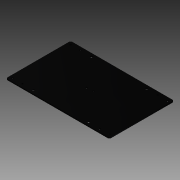
# Autodesk Inventor part: y-carriage
Saved by Autodesk Inventor 2014 (Build 180170000, 170)
## iProperties
Created: 2013-07-12
Part Number: y-carriage
Material: Steel, Mild
Document SubType Name: Modeling
Designer: Edward
Density: 7.86 g/cm^3
Appearance: Smooth - Black
Author: Edward
Autodesk Inventor part; units mm, degrees
ref_plane "YZ Plane" through (0, 0, 0) normal (1, 0, 0) x (0, 1, 0)
ref_plane "XZ Plane" through (0, 0, 0) normal (0, 1, 0) x (-1, 0, 0)
ref_plane "XY Plane" through (0, 0, 0) normal (0, 0, 1) x (1, 0, 0)
sketch "Sketch1" plane through (0, 0, 0) normal (0, 0, 1) x (1, 0, 0)
  line L0 (-160, 100) -> (160, 100)
  line L1 (160, 100) -> (160, -100)
  line L2 (160, -100) -> (-160, -100)
  line L3 (-160, -100) -> (-160, 100)
  point P0 (0, 0)
  dimension "d0" = 320
  dimension "d1" = 200
  dimension "d2" = 160
  dimension "d3" = 100
  constraints: 8 end point, 2 parallel, 1 horizontal, 1 perpendicular
  measures "d0" distance of L1.end L2.end
  measures "d1" distance of L0.end L1.end
  measures "d2" distance from line of point (0, 0) L3
  measures "d3" distance from line of L0 point (0, 0)
extrude "Extrusion1" add sketch "Sketch1" along normal blind 3.4163
sketch "Sketch2" plane through (0, 0, 3.4163) normal (0, 0, 1) x (1, 0, 0)
  line L0 (160, 100) -> (-160, 100) projected
  line L1 (-160, 100) -> (-160, -100) projected
  line L2 (-160, -100) -> (160, -100) projected
  line L3 (160, -100) -> (160, 100) projected
  circle A0 centre (-150, -90) radius 2.75
  circle A1 centre (-150, 90) radius 2.75
  circle A2 centre (-85.4, 90) radius 3.58
  circle A3 centre (-85.4, -90) radius 3.58
  circle A4 centre (85.4, 90) radius 3.58
  circle A5 centre (150, 90) radius 2.75
  circle A6 centre (85.4, -90) radius 3.58
  circle A7 centre (150, -90) radius 2.75
  point P0 (0, 0)
  dimension "d6" = 5.5
  dimension "d7" = 5.5
  dimension "d8" = 7.16
  dimension "d9" = 7.16
  dimension "d10" = 7.16
  dimension "d11" = 5.5
  dimension "d12" = 7.16
  dimension "d13" = 5.5
  dimension "d14" = 10
  dimension "d15" = 10
  dimension "d16" = 64.6
  dimension "d17" = 10
  dimension "d18" = 64.6
  dimension "d19" = 10
  dimension "d20" = 10
  dimension "d21" = 10
  dimension "d22" = 10
  dimension "d23" = 10
  dimension "d24" = 10
  dimension "d25" = 10
  dimension "d26" = 10
  dimension "d27" = 64.6
  dimension "d28" = 64.6
  dimension "d29" = 10
  constraints: 8 centre point
  measures "d6" diameter of A0
  measures "d7" diameter of A1
  measures "d8" diameter of A2
  measures "d9" diameter of A3
  measures "d10" diameter of A4
  measures "d11" diameter of A5
  measures "d12" diameter of A6
  measures "d13" diameter of A7
  measures "d14" distance from line of L2 A0.centre
  measures "d15" distance from line of L1 A0.centre
  measures "d16" distance of A3.centre A0.centre
  measures "d17" distance from line of L2 A3.centre
  measures "d18" distance of A2.centre A1.centre
  measures "d19" distance from line of L0 A1.centre
  measures "d20" distance from line of L1 A1.centre
  measures "d21" distance from line of L0 A2.centre
  measures "d22" distance from line of L2 A7.centre
  measures "d23" distance from line of L3 A7.centre
  measures "d24" distance from line of L3 A5.centre
  measures "d25" distance from line of L0 A5.centre
  measures "d26" distance from line of L0 A4.centre
  measures "d27" distance of A5.centre A4.centre
  measures "d28" distance of A6.centre A7.centre
  measures "d29" distance from line of L2 A6.centre
extrude "Extrusion2" cut sketch "Sketch2" against normal through all contours A0 | A1 | A2 | A3 | A4 | A5 | A6 | A7
fillet "Fillet1" radius 5 4 edges at (-160, -100, 1.7082) (-160, 100, 1.7082) (160, 100, 1.7082) (160, -100, 1.7082)
sketch "Sketch3" plane through (0, 0, 0) normal (0, 0, -1) x (-1, 0, 0)
  circle A0 centre (-10, 0) radius 2.067 projected
  circle A1 centre (10, 0) radius 2.067 projected
  circle A2 centre (-10, 0) radius 2.75
  circle A3 centre (10, 0) radius 2.75
  point P0 (0, 0)
  dimension "d33" = 5.5
  dimension "d34" = 5.5
  constraints: 2 centre point, 2 coincident
  measures "d33" diameter of A2
  measures "d34" diameter of A3
extrude "Extrusion3" cut sketch "Sketch3" against normal through all contours A0 | A1 | A2 | A3
sketch "Sketch4" plane through (0, 0, 0) normal (0, 0, -1) x (-1, 0, 0)
  line L0 (-155, -100) -> (155, -100) projected
  line L1 (-160, 95) -> (-160, -95) projected
  circle A0 centre (-120, -90) radius 2.75
  point P0 (0, 0)
  dimension "d37" = 5.5
  dimension "d38" = 40
  dimension "d39" = 10
  constraints: 1 centre point
  measures "d37" diameter of A0
  measures "d38" distance from line of L1 A0.centre
  measures "d39" distance from line of L0 A0.centre
extrude "Extrusion4" cut sketch "Sketch4" against normal through all
pattern_linear "Rectangular Pattern1" count 2 spacing 240 along (-1, 0, 0) count 2 spacing 180 along (0, 1, 0) of "Extrusion4"
equation "\"d2\" = 0.5 * d0"
equation "\"d3\" = 0.5 * d1"
body "Solid1"
